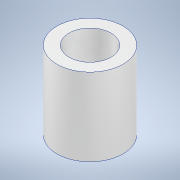
# Autodesk Inventor part: gearbox to waterjoint coupling
Saved by Autodesk Inventor 2021 (Build 250183000, 183)
## iProperties
Created: 2021-03-29
Part Number: gearbox to waterjoint coupling
Material: Aluminum 6061
Document SubType Name: Modeling
Designer: Work
Mass: 13.6924 g
Surface Area: 27.9499 cm^2
Volume: 5.07124 cm^3
Density: 2.7 g/cm^3
Appearance: Aluminum - Flat
Author: Work
Autodesk Inventor part; units mm, degrees
ref_plane "YZ Plane" through (0, 0, 0) normal (1, 0, 0) x (0, 1, 0)
ref_plane "XZ Plane" through (0, 0, 0) normal (0, 1, 0) x (-1, 0, 0)
ref_plane "XY Plane" through (0, 0, 0) normal (0, 0, 1) x (1, 0, 0)
sketch "Sketch1" plane through (0, 0, 0) normal (1, 0, 0) x (0, 1, 0)
  line L0 (1, 4.5) -> (10.5, 4.5)
  line L1 (10.5, 4.5) -> (10.5, 6.35)
  line L2 (10.5, 6.35) -> (23.5175, 6.35)
  line L3 (23.5175, 6.35) -> (23.5175, 10)
  line L4 (23.5175, 10) -> (0, 10)
  line L5 (0, 10) -> (0, 5.05)
  line L6 (-4.7035, 0) -> (28.221, 0) projected
  line L7 (0, 5.05) -> (0, 4.5)
  line L8 (0, 4.5) -> (1, 4.5)
  point P0 (0, 0)
  dimension "d1" = 4.5
  dimension "d2" = 6.35
  dimension "d3" = 10
  dimension "d5" = 10.5
  dimension "d6" = 13.0175
  constraints: 16 end point, 7 perpendicular, 1 point on line
  measures "d1" distance from line of point (0, 0) L0
  measures "d2" distance from line of point (0, 0) L2
  measures "d3" distance from line of point (0, 0) L4
  measures "d5" distance between parallel lines of L5 L1
  measures "d6" distance between parallel lines of L1 L3
revolve "Revolution1" add sketch "Sketch1" angle 360 about axis through (0, -10, 0) along (0, 1, 0)
body "Solid1"
